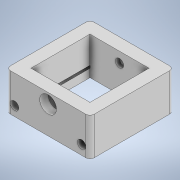
# Autodesk Inventor part: Деталь3
Saved by Autodesk Inventor 2020.2 (Build 242310000, 310)
## iProperties
Created: 2026-03-04
Part Number: Деталь3
Material: Типовые
Document SubType Name: Modeling
Designer: tankfpv
Density: 1 g/cm^3
Appearance: По умолчанию
Author: tankfpv
Autodesk Inventor part; units mm, degrees
ref_plane "YZ Plane" through (0, 0, 0) normal (1, 0, 0) x (0, 1, 0)
ref_plane "XZ Plane" through (0, 0, 0) normal (0, 1, 0) x (-1, 0, 0)
ref_plane "XY Plane" through (0, 0, 0) normal (0, 0, 1) x (1, 0, 0)
sketch "Эскиз1" plane through (0, 0, 0) normal (0, 1, 0) x (-1, 0, 0)
  line L0 (7.05, -7.05) -> (-7.05, -7.05)
  line L1 (-7.05, -7.05) -> (-7.05, 7.05)
  line L2 (-7.05, 7.05) -> (7.05, 7.05)
  line L3 (7.05, 7.05) -> (7.05, -7.05)
  line L4 (7.05, -7.05) -> (-7.05, 7.05) construction
  line L5 (-7.05, -7.05) -> (7.05, 7.05) construction
  line L6 (-10, -10) -> (10, -10)
  line L7 (10, -10) -> (10, 10)
  line L8 (10, 10) -> (-10, 10)
  line L9 (-10, 10) -> (-10, -10)
  line L10 (-10, -10) -> (10, 10) construction
  line L11 (10, -10) -> (-10, 10) construction
  point P0 (0, 0)
  dimension "d0" = 14.1
  dimension "d1" = 14.1
  dimension "d2" = 20
  dimension "d3" = 20
  constraints: 24 end point, 4 midpoint, 4 parallel, 2 horizontal, 2 perpendicular
  measures "d0" distance of L1.end L2.end
  measures "d1" distance of L0.end L1.end
  measures "d2" distance of L8.end L7.end
  measures "d3" distance of L7.end L6.end
extrude "Выдавливание1" add sketch "Эскиз1" along normal blind 9
sketch "Эскиз2" plane through (-10, 0, 10) normal (0, 0, 1) x (1, 0, 0)
  line L0 (0, 0) -> (0, 9) projected
  line L1 (20, 9) -> (0, 9) projected
  line L2 (0, 0) -> (20, 9)
  line L3 (0, 9) -> (20, 0)
  line L4 (0, 4.5) -> (20, 4.5)
  line L5 (20, 0) -> (0, 0) projected
  line L6 (20, 4.5) -> (0, 0)
  line L7 (0, 4.5) -> (20, 0)
  line L8 (10, 2.25) -> (2, 2.25)
  line L9 (2, 2.25) -> (18, 2.25)
  circle A0 centre (2, 2.25) radius 1
  circle A1 centre (18, 2.25) radius 1
  circle A2 centre (10, 6.5217) radius 1
  circle A3 centre (10, 6.5217) radius 2
  point P0 (10, 0)
  dimension "d6" = 8
  dimension "d7" = 16
  dimension "d8" = 2
  dimension "d9" = 2
  dimension "d10" = 2
  dimension "d11" = 4
  constraints: 14 end point, 4 centre point, 3 coincident, 2 horizontal, 2 midpoint, 1 point on line
  measures "d6" distance of L8.start L8.end
  measures "d7" distance of L8.end L9.end
  measures "d8" diameter of A0
  measures "d9" diameter of A1
  measures "d10" diameter of A2
  measures "d11" diameter of A3
sketch "Эскиз3" plane through (-10, 0, 10) normal (0, 0, 1) x (1, 0, 0)
  circle A0 centre (10, 6.5383) radius 2
  point P0 (10, 0)
  dimension "d12" = 4
  constraints: 1 centre point
  measures "d12" diameter of A0
extrude "Выдавливание2" cut sketch "Эскиз2" against normal blind 25 contours A1 | A0 | A2
sketch "Эскиз4" plane through (10, 0, -10) normal (0, 0, -1) x (-1, 0, 0)
  circle A0 centre (10, 6.5217) radius 1 projected
  circle A1 centre (10, 6.5217) radius 2
  point P0 (10, 0)
  dimension "d15" = 4
  constraints: 1 centre point, 1 coincident
  measures "d15" diameter of A1
extrude "Выдавливание3" cut sketch "Эскиз3" against normal blind 2
extrude "Выдавливание4" cut sketch "Эскиз4" against normal blind 2
fillet "Сопряжение1" radius 1 4 edges at (-10, 4.5, 10) (10, 4.5, 10) (10, 4.5, -10) (-10, 4.5, -10)
